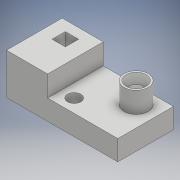
# Autodesk Inventor part: Part3
Saved by Autodesk Inventor 2018 (Build 220112000, 112)
## iProperties
Created: 2017-11-09
Part Number: Part3
Material: Generic
Document SubType Name: Modeling
Designer: kurtis
Density: 1 g/cm^3
Appearance: Default
Author: kurtis
Autodesk Inventor part; units mm, degrees
ref_plane "YZ Plane" through (0, 0, 0) normal (1, 0, 0) x (0, 1, 0)
ref_plane "XZ Plane" through (0, 0, 0) normal (0, 1, 0) x (-1, 0, 0)
ref_plane "XY Plane" through (0, 0, 0) normal (0, 0, 1) x (1, 0, 0)
sketch "Sketch1" plane through (0, 0, 0) normal (0, 0, 1) x (1, 0, 0)
  line L0 (0, 0) -> (16.25, 0)
  line L1 (44, 0) -> (44, 22)
  line L2 (44, 22) -> (16.25, 22)
  line L3 (0, 22) -> (0, 0)
  line L4 (5.25, 18) -> (10.5, 18)
  line L5 (10.5, 18) -> (10.5, 12.75)
  line L6 (10.5, 12.75) -> (5.25, 12.75)
  line L7 (5.25, 12.75) -> (5.25, 18)
  line L8 (16.25, 22) -> (16.25, 0)
  line L9 (16.25, 22) -> (0, 22)
  line L10 (16.25, 0) -> (44, 0)
  circle A0 centre (21.5, 5.25) radius 2.625
  circle A1 centre (36, 15.25) radius 4.75
  circle A2 centre (36, 15.25) radius 4
  circle A3 centre (36, 15.25) radius 2.625
  dimension "d0" = 44
  dimension "d1" = 22
  dimension "d2" = 5.25
  dimension "d3" = 5.25
  dimension "d4" = 16.25
  dimension "d5" = 5.25
  dimension "d6" = 5.25
  dimension "d7" = 5.25
  dimension "d8" = 4
  dimension "d9" = 5.25
  dimension "d10" = 6.75
  dimension "d11" = 8
  dimension "d12" = 5.25
  dimension "d13" = 8
  dimension "d14" = 9.5
  constraints: 22 end point, 7 parallel, 5 perpendicular, 4 centre point, 3 horizontal, 2 coincident
  measures "d0" distance of L3.start L1.end
  measures "d1" distance of L1.end L1.start
  measures "d2" distance of L5.end L6.end
  measures "d3" distance of L4.end L5.end
  measures "d4" distance between parallel lines of L8 L3
  measures "d5" distance from line of L10 A0.centre
  measures "d6" distance from line of L8 A0.centre
  measures "d7" diameter of A0
  measures "d8" distance between parallel lines of L9 L4
  measures "d9" distance between parallel lines of L3 L7
  measures "d10" distance from line of L2 A1.centre
  measures "d11" distance from line of A1.centre L1
  measures "d12" diameter of A3
  measures "d13" diameter of A2
  measures "d14" diameter of A1
extrude "Extrusion1" add sketch "Sketch1" along normal blind 8 contours L3 L9 L8 L0 | L8 L2 L1 L10 | A1 | A2 | A3
extrude "Extrusion2" add sketch "Sketch1" along normal blind 16.25 contours L3 L9 L8 L0 | A1
extrude "Extrusion3" add sketch "Sketch1" along normal blind 13 contours A2 | A3
chamfer "Chamfer1" distance 3.25 distance2 1.25 1 edges at (32, 15.25, 13) measured on face at (39.987, 14.9281, 15.1667)
body "Solid1"
